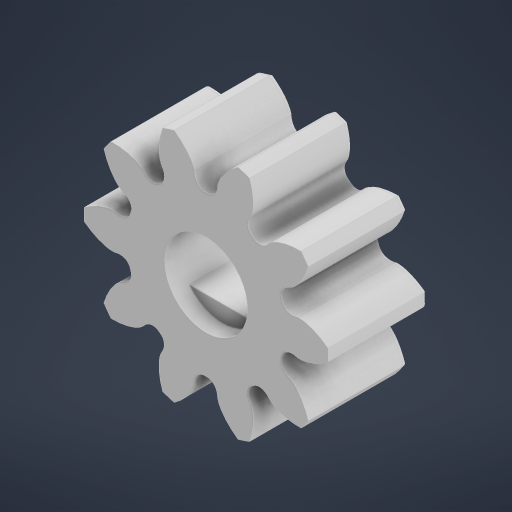
# Autodesk Inventor part: pinion
Saved by Autodesk Inventor 2024 (Build 280153000, 153)
## iProperties
Created: 2024-05-11
Part Number: pinion
Material: Generic
Document SubType Name: Modeling
Designer: loren
Density: 1 g/cm^3
Appearance: Default
Author: loren
## iProperties of the stored document pinion_3DPrint.ipt
Created: 2026-02-06
Part Number: pinion_3DPrint
Material: Generic
Document SubType Name: Modeling
Designer: lokies
Density: 1 g/cm^3
Appearance: Default
Author: lokies
Autodesk Inventor part; units mm, degrees
ref_plane "YZ Plane" through (0, 0, 0) normal (1, 0, 0) x (0, 1, 0)
ref_plane "XZ Plane" through (0, 0, 0) normal (0, 1, 0) x (-1, 0, 0)
ref_plane "XY Plane" through (0, 0, 0) normal (0, 0, 1) x (1, 0, 0)
sketch "Sketch1" plane through (0, 0, 0) normal (0, 0, 1) x (1, 0, 0)
  spline S0 degree 3 poles (-1.9189, 7.091) (-1.8526, 7.0433) (-1.7202, 6.9479) (-1.532, 6.7909) (-1.353, 6.6237) (-1.2134, 6.4747) (-1.1084, 6.3497) (-1.0334, 6.2528) (-0.9626, 6.1529) (-0.8965, 6.0499) (-0.8356, 5.9435) (-0.7816, 5.8337) (-0.7339, 5.7206) (-0.7137, 5.6415) (-0.7037, 5.6019) knots 0 0 0 0 0.024484 0.048967 0.07345 0.097933 0.110176 0.122418 0.134661 0.146903 0.159145 0.171387 0.183627 0.195858 0.195858 0.195858 0.195858
  spline S1 degree 3 poles (-0.7037, 5.6019) (-0.701, 5.5508) (-0.6969, 5.4742) (-0.6811, 5.373) (-0.6633, 5.2984) (-0.6416, 5.2247) (-0.6127, 5.1535) (-0.5778, 5.0851) (-0.5362, 5.0206) (-0.4874, 4.9612) (-0.4317, 4.9081) (-0.3693, 4.8632) (-0.3013, 4.8272) (-0.2289, 4.8016) (-0.1284, 4.7799) (0, 4.7878) (0.1284, 4.7799) (0.2289, 4.8016) (0.3013, 4.8272) (0.3693, 4.8632) (0.4317, 4.9081) (0.4874, 4.9612) (0.5362, 5.0206) (0.5778, 5.0851) (0.6127, 5.1535) (0.6416, 5.2247) (0.6633, 5.2984) (0.6811, 5.373) (0.6969, 5.4742) (0.701, 5.5508) (0.7037, 5.6019) knots 0 0 0 0 0.015336 0.023007 0.030677 0.038347 0.046017 0.053685 0.061352 0.06902 0.07669 0.084358 0.092023 0.099684 0.107352 0.122686 0.138021 0.145689 0.15335 0.161014 0.168683 0.176353 0.184021 0.191688 0.199355 0.207026 0.214696 0.222366 0.230037 0.245373 0.245373 0.245373 0.245373
  spline S2 degree 3 poles (0.7037, 5.6019) (0.7137, 5.6415) (0.7339, 5.7206) (0.7816, 5.8337) (0.8356, 5.9435) (0.8965, 6.0499) (0.9626, 6.1529) (1.0334, 6.2528) (1.1084, 6.3497) (1.2134, 6.4747) (1.353, 6.6237) (1.532, 6.7909) (1.7202, 6.9479) (1.8526, 7.0433) (1.9189, 7.091) knots 0 0 0 0 0.012231 0.024471 0.036713 0.048955 0.061197 0.07344 0.085683 0.097926 0.122408 0.146891 0.171375 0.195858 0.195858 0.195858 0.195858
  circle A0 centre (0, 0) radius 4.7846 construction
  circle A1 centre (0, 0) radius 5.6382 construction
  circle A2 centre (0, 0) radius 6 construction
  circle A3 centre (0, 0) radius 7.3461
  point P0 (-1.7219, 6.9456)
  point P1 (-1.5335, 6.7892)
  point P2 (-1.3549, 6.6218)
  point P3 (-1.1877, 6.443)
  point P4 (-1.109, 6.3491)
  point P5 (-1.0341, 6.2523)
  point P6 (-0.9634, 6.1524)
  point P7 (-0.8973, 6.0493)
  point P8 (-0.8368, 5.9429)
  point P9 (-0.7827, 5.8331)
  point P10 (-0.7368, 5.7196)
  point P11 (-0.6921, 5.449)
  point P12 (-0.6801, 5.3732)
  point P13 (-0.6626, 5.2985)
  point P14 (-0.6404, 5.2251)
  point P15 (-0.6117, 5.154)
  point P16 (-0.5767, 5.0858)
  point P17 (-0.535, 5.0214)
  point P18 (-0.4863, 4.9622)
  point P19 (-0.4306, 4.9095)
  point P20 (-0.3684, 4.8647)
  point P21 (-0.3006, 4.8289)
  point P22 (-0.2284, 4.8031)
  point P23 (-0.1533, 4.7877)
  point P24 (0, 4.7846)
  point P25 (0.1533, 4.7877)
  point P26 (0.2284, 4.8031)
  point P27 (0.3006, 4.8289)
  point P28 (0.3684, 4.8647)
  point P29 (0.4306, 4.9095)
  point P30 (0.4863, 4.9622)
  point P31 (0.535, 5.0214)
  point P32 (0.5767, 5.0858)
  point P33 (0.6117, 5.154)
  point P34 (0.6404, 5.2251)
  point P35 (0.6626, 5.2985)
  point P36 (0.6801, 5.3732)
  point P37 (0.6921, 5.449)
  point P38 (0.7368, 5.7196)
  point P39 (0.7827, 5.8331)
  point P40 (0.8368, 5.9429)
  point P41 (0.8973, 6.0493)
  point P42 (0.9634, 6.1524)
  point P43 (1.0341, 6.2523)
  point P44 (1.109, 6.3491)
  point P45 (1.1877, 6.443)
  point P46 (1.3549, 6.6218)
  point P47 (1.5335, 6.7892)
  point P48 (1.7219, 6.9456)
  constraints: 4 centre point, 2 point on circle, 113 other
extrude "Extrusion1" add sketch "Sketch1" against normal blind 6
extrude "Extrusion2" cut sketch "Sketch1" against normal through all contours A3 S2 S1 S0 picked at (0.2088, 6.3635)
pattern_circular "Circular Pattern1" count 10 over 360 about axis through (0, 0, -10) along (0, 0, 1) of "Extrusion2"
sketch "Sketch2" plane through (0, 0, 0) normal (0, 0, 1) x (1, 0, 0)
  line L0 (-2, 1.5) -> (2, 1.5)
  line L1 (-2, -1.5) -> (2, -1.5)
  circle A0 centre (0, 0) radius 2.5
  dimension "d8" = 3
  dimension "d15" = 5
  constraints: 4 end point, 4 point on circle, 2 horizontal, 1 centre point, 1 coincident, 1 parallel
  measures "d8" distance between parallel lines of L1 L0
  measures "d15" diameter of A0
extrude "Extrusion3" cut sketch "Sketch2" against normal through all contours L0 A0 L1
extrude "Extrusion4" cut sketch "Sketch2" against normal blind 1 contours A0 L0 | L1 A0
fillet "Fillet1" radius 0.3 40 edges at (4.748, 4.5144, -6) (5.9431, 4.3179, -6) (5.7606, 3.1206, -6) (4.5504, 1.4786, -6) (6.4947, 0.8614, -6) (7.3461, 0, -6) (6.4947, -0.8614, -6) (4.5505, -1.4785, -6) (5.7606, -3.1206, -6) (5.9431, -4.3179, -6) (4.748, -4.5144, -6) (2.8124, -3.8708, -6) (2.8262, -5.9106, -6) (2.2701, -6.9866, -6) (1.1877, -6.443, -6) (0.0001, -4.7846, -6) (-1.1877, -6.443, -6) (-2.2701, -6.9866, -6) (-2.8262, -5.9106, -6) (-2.8123, -3.8709, -6) (-4.748, -4.5144, -6) (-5.9431, -4.3179, -6) (-5.7606, -3.1206, -6) (-4.5504, -1.4786, -6) (-6.4947, -0.8614, -6) (-7.3461, 0, -6) (-6.4947, 0.8614, -6) (-4.5505, 1.4785, -6) (-5.7606, 3.1206, -6) (-5.9431, 4.3179, -6) (-4.748, 4.5144, -6) (-2.8124, 3.8708, -6) (-2.8262, 5.9106, -6) (-2.2701, 6.9866, -6) (-1.1877, 6.443, -6) (-0.0001, 4.7846, -6) (1.1877, 6.443, -6) (2.2701, 6.9866, -6) (2.8262, 5.9106, -6) (2.8123, 3.8709, -6)
equation "\"Module\" = 1.2"
equation "\"PressureAngle\" = 20deg"
equation "\"UnitProfileClearance\" = 0.25"
equation "\"UnitRoundRadius\" = 0.35"
equation "\"HeadDiameter\" = 14.69219"
equation "\"RootDiameter\" = 9.56927"
equation "\"BaseDiameter\" = 11.27631"
equation "\"PitchDiameter\" = 12"
equation "\"FaceWidth\" = 5"
equation "\"HelixAngle\" = 0"
equation "\"UnitCorrection\" = 0.237196"
equation "\"UnitAddendumModification\" = 0.115452"
equation "\"CircularPitch\" = 3.76991"
equation "\"UnitBacklashShift\" = 0"
equation "\"TotalToolShift\" = 0.28464"
equation "\"IsInternal\" = 0"
equation "\"elephant_prevention_radius\" = 0.3"
body "Solid1"
